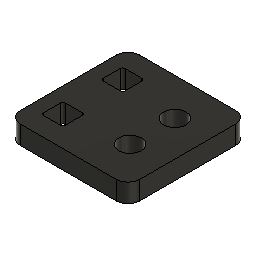
Load Cell Mount (Autodesk Fusion 360 design; units mm, degrees)
Autodesk Fusion 360 part; units mm, degrees
sketch "Sketch1" plane through (-0.0003, 0, -14.0546) normal (0.000019, 0, 1) x (0, 1, 0)
  arc A0 (15.0114, -7.5039) -> (14.5034, -6.9959) centre (14.5034, -7.5039) ccw
  line L0 (15.0114, -7.5039) -> (15.0114, -11.1107)
  arc A1 (14.5034, -11.6187) -> (15.0114, -11.1107) centre (14.5034, -11.1107) ccw
  line L1 (14.5034, -11.6187) -> (10.8966, -11.6187)
  arc A2 (10.3886, -11.1107) -> (10.8966, -11.6187) centre (10.8966, -11.1107) ccw
  line L2 (10.3886, -11.1107) -> (10.3886, -7.5039)
  arc A3 (10.8966, -6.9959) -> (10.3886, -7.5039) centre (10.8966, -7.5039) ccw
  line L3 (10.8966, -6.9959) -> (14.5034, -6.9959)
  arc A4 (27.7114, -7.5039) -> (27.2034, -6.9959) centre (27.2034, -7.5039) ccw
  line L4 (27.7114, -7.5039) -> (27.7114, -11.1107)
  arc A5 (27.2034, -11.6187) -> (27.7114, -11.1107) centre (27.2034, -11.1107) ccw
  line L5 (27.2034, -11.6187) -> (23.5966, -11.6187)
  arc A6 (23.0886, -11.1107) -> (23.5966, -11.6187) centre (23.5966, -11.1107) ccw
  line L6 (23.0886, -11.1107) -> (23.0886, -7.5039)
  arc A7 (23.5966, -6.9959) -> (23.0886, -7.5039) centre (23.5966, -7.5039) ccw
  line L7 (23.5966, -6.9959) -> (27.2034, -6.9959)
  arc A8 (40.4114, -7.5039) -> (39.9034, -6.9959) centre (39.9034, -7.5039) ccw
  line L8 (40.4114, -7.5039) -> (40.4114, -11.1107)
  arc A9 (39.9034, -11.6187) -> (40.4114, -11.1107) centre (39.9034, -11.1107) ccw
  line L9 (39.9034, -11.6187) -> (36.2966, -11.6187)
  arc A10 (35.7886, -11.1107) -> (36.2966, -11.6187) centre (36.2966, -11.1107) ccw
  line L10 (35.7886, -11.1107) -> (35.7886, -7.5039)
  arc A11 (36.2966, -6.9959) -> (35.7886, -7.5039) centre (36.2966, -7.5039) ccw
  line L11 (36.2966, -6.9959) -> (39.9034, -6.9959)
  arc A12 (53.1114, -7.5039) -> (52.6034, -6.9959) centre (52.6034, -7.5039) ccw
  line L12 (53.1114, -7.5039) -> (53.1114, -11.1107)
  arc A13 (52.6034, -11.6187) -> (53.1114, -11.1107) centre (52.6034, -11.1107) ccw
  line L13 (52.6034, -11.6187) -> (48.9966, -11.6187)
  arc A14 (48.4886, -11.1107) -> (48.9966, -11.6187) centre (48.9966, -11.1107) ccw
  line L14 (48.4886, -11.1107) -> (48.4886, -7.5039)
  arc A15 (48.9966, -6.9959) -> (48.4886, -7.5039) centre (48.9966, -7.5039) ccw
  line L15 (48.9966, -6.9959) -> (52.6034, -6.9959)
  arc A16 (65.8114, -7.5039) -> (65.3034, -6.9959) centre (65.3034, -7.5039) ccw
  line L16 (65.8114, -7.5039) -> (65.8114, -11.1107)
  arc A17 (65.3034, -11.6187) -> (65.8114, -11.1107) centre (65.3034, -11.1107) ccw
  line L17 (65.3034, -11.6187) -> (61.6966, -11.6187)
  arc A18 (61.1886, -11.1107) -> (61.6966, -11.6187) centre (61.6966, -11.1107) ccw
  line L18 (61.1886, -11.1107) -> (61.1886, -7.5039)
  arc A19 (61.6966, -6.9959) -> (61.1886, -7.5039) centre (61.6966, -7.5039) ccw
  line L19 (61.6966, -6.9959) -> (65.3034, -6.9959)
  arc A20 (2.3114, -7.5039) -> (1.8034, -6.9959) centre (1.8034, -7.5039) ccw
  line L20 (2.3114, -7.5039) -> (2.3114, -11.1107)
  arc A21 (1.8034, -11.6187) -> (2.3114, -11.1107) centre (1.8034, -11.1107) ccw
  line L21 (1.8034, -11.6187) -> (-1.8034, -11.6187)
  arc A22 (-2.3114, -11.1107) -> (-1.8034, -11.6187) centre (-1.8034, -11.1107) ccw
  line L22 (-2.3114, -11.1107) -> (-2.3114, -7.5039)
  arc A23 (-1.8034, -6.9959) -> (-2.3114, -7.5039) centre (-1.8034, -7.5039) ccw
  line L23 (-1.8034, -6.9959) -> (1.8034, -6.9959)
  line L24 (69.85, -15.6573) -> (69.85, -4.1003)
  line L25 (69.85, -4.1003) -> (58.1488, -4.1003)
  line L26 (58.1488, -4.1003) -> (57.15, -5.0991)
  line L27 (57.15, -5.0991) -> (56.1512, -4.1003)
  line L28 (56.1512, -4.1003) -> (-6.35, -4.1003)
  line L29 (-6.35, -4.1003) -> (-6.35, -13.1692)
  arc A24 (-6.35, -13.1692) -> (-6.2036, -13.5228) centre (-5.85, -13.1692) ccw
  line L30 (-6.2036, -13.5228) -> (-4.2155, -15.5109)
  arc A25 (-4.2155, -15.5109) -> (-3.8619, -15.6573) centre (-3.8619, -15.1573) ccw
  line L31 (-3.8619, -15.6573) -> (54.6619, -15.6573)
  arc A26 (54.6619, -15.6573) -> (55.0155, -15.5109) centre (54.6619, -15.1573) ccw
  line L32 (55.0155, -15.5109) -> (56.7964, -13.7299)
  arc A27 (57.5036, -13.7299) -> (56.7964, -13.7299) centre (57.15, -14.0834) ccw
  line L33 (57.5036, -13.7299) -> (59.2845, -15.5109)
  arc A28 (59.2845, -15.5109) -> (59.6381, -15.6573) centre (59.6381, -15.1573) ccw
  line L34 (59.6381, -15.6573) -> (69.85, -15.6573)
  line L35 (69.85, -6.6403) -> (69.85, -26.9603)
  line L36 (67.31, -29.5003) -> (46.99, -29.5003)
  line L37 (44.45, -26.9603) -> (44.45, -6.6403)
  line L38 (46.99, -4.1003) -> (67.31, -4.1003)
  arc A29 (46.99, -4.1003) -> (44.45, -6.6403) centre (46.99, -6.6403) ccw
  arc A30 (69.85, -6.6403) -> (67.31, -4.1003) centre (67.31, -6.6403) ccw
  arc A31 (67.31, -29.5003) -> (69.85, -26.9603) centre (67.31, -26.9603) ccw
  arc A32 (44.45, -26.9603) -> (46.99, -29.5003) centre (46.99, -26.9603) ccw
  line L39 (69.85, -15.6573) -> (69.85, -22.0073)
  line L40 (69.85, -22.0073) -> (44.45, -22.0073)
  line L41 (69.85, -22.0073) -> (61.9125, -22.0073)
  circle A33 centre (61.9125, -22.0073) radius 2.3813
  line L42 (61.9125, -22.0073) -> (52.3875, -22.0073)
  circle A34 centre (52.3875, -22.0073) radius 2.3813
  point P0 (69.85, -4.1003)
  point P1 (69.85, -29.5003)
  point P2 (44.45, -29.5003)
  point P3 (44.45, -4.1003)
  dimension "d1" = 25.4
  dimension "d2" = 25.4
  dimension "d3" = 25.4
  dimension "d4" = 2.54
  dimension "d5" = 6.35
  dimension "d6" = 7.9375
  dimension "d7" = 4.7625
  dimension "d8" = 9.525
  dimension "d9" = 4.7625
  constraint coincident P0 L24.end
  constraint perpendicular L25 L35
  constraint perpendicular L24 L36
  constraint perpendicular L28 L37
  constraint coincident P3 L37
  constraint coincident P3 L38
  constraint tangent L37 A29
  constraint tangent L38 A29
  constraint coincident P0 L35
  constraint coincident P0 L38
  constraint tangent L35 A30
  constraint tangent L38 A30
  constraint equal A29 A30
  constraint coincident P1 L35
  constraint coincident P1 L36
  constraint tangent L35 A31
  constraint tangent L36 A31
  constraint equal A29 A31
  constraint coincident P2 L36
  constraint coincident P2 L37
  constraint tangent L36 A32
  constraint tangent L37 A32
  constraint equal A29 A32
  constraint coincident L24.start L34.end
  constraint coincident L35 L39.end
  constraint coincident L37 L40.end
  constraint perpendicular L37 L40
  constraint coincident L40 L41.end
  constraint coincident L41.end A33.centre
  constraint coincident L40 L42.end
  constraint coincident L42.end A34.centre
  measures "d1" distance of P0 P1
  measures "d2" distance of P1 P2
  measures "d3" distance of P2 P3
  measures "d4" radius of A29
  measures "d5" distance of L24.start L39.end
  measures "d6" distance of L39.end L41.end
  measures "d7" diameter of A33
  measures "d8" distance of L41.end L42.end
  measures "d9" diameter of A34
extrude "Extrude1" add sketch "Sketch1" along normal blind 3.9688 contours L24 L25 L26 L27 L28 L31 A26 L32 A27 L33 A28 L34 L35 L37 L38 A29 A30 | L31 A26 L32 A27 L33 A28 L34 L35 L37 L39 L40 L41 A33 L42 A34 | L35 L36 L37 A31 A32 L40 L41 A33 L42 A34 | L26 L27 L38
equation "d5 = ( 1 / 4 ) * 1 in"
equation "d6 = ( 5 / 16 ) * 1 in"
equation "d7 = ( 3 / 16 ) * 1 in"
equation "d8 = ( 3 / 8 ) * 1 in"
equation "d9 = ( 3 / 16 ) * 1 in"
equation "d10 = ( 5 / 32 ) * 1 in"
named bodies: "LoadCellMount"
